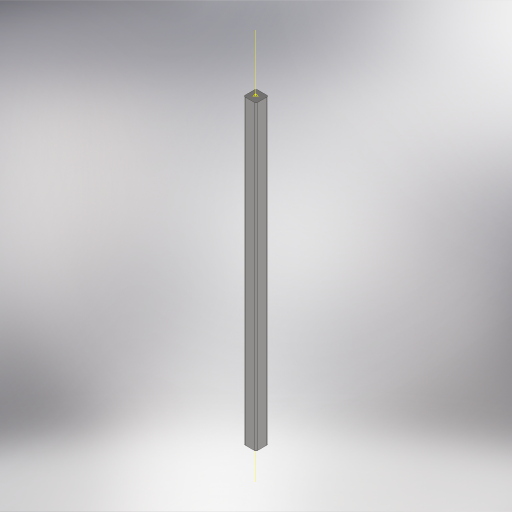
# Autodesk Inventor part: LS-Shaft-3.00in
Saved by Autodesk Inventor 2023 (Build 270158000, 158)
## iProperties
Created: 2023-01-31
Part Number: LS-Shaft-3.00in
Material: Stainless Steel
Document SubType Name: Modeling
Designer: aaron
Density: 8 g/cm^3
Appearance: Semi-Polished
Author: aaron
Autodesk Inventor part; units mm, degrees
ref_plane "YZ Plane" through (0, 0, 0) normal (1, 0, 0) x (0, 1, 0)
ref_plane "XZ Plane" through (0, 0, 0) normal (0, 1, 0) x (-1, 0, 0)
ref_plane "XY Plane" through (0, 0, 0) normal (0, 0, 1) x (1, 0, 0)
sketch "Sketch1" plane through (0, 0, 0) normal (0, 1, 0) x (-1, 0, 0)
  line L0 (-1.5875, -1.5875) -> (1.5875, -1.5875)
  line L1 (1.5875, -1.5875) -> (1.5875, 1.5875)
  line L2 (1.5875, 1.5875) -> (-1.5875, 1.5875)
  line L3 (-1.5875, 1.5875) -> (-1.5875, -1.5875)
  line L4 (-1.5875, -1.5875) -> (1.5875, 1.5875) construction
  line L5 (1.5875, -1.5875) -> (-1.5875, 1.5875) construction
  point P0 (0, 0)
  dimension "d0" = 3.175
  dimension "d1" = 3.175
  constraints: 12 end point, 2 midpoint, 2 parallel, 1 horizontal, 1 perpendicular
  measures "d0" distance of L2.end L1.end
  measures "d1" distance of L1.end L0.end
extrude "Extrusion1" add sketch "Sketch1" along normal blind 76.2
fillet "Fillet1" radius 0.3969 4 edges at (1.5875, 38.1, 1.5875) (1.5875, 38.1, -1.5875) (-1.5875, 38.1, -1.5875) (-1.5875, 38.1, 1.5875)
body "Solid1"
